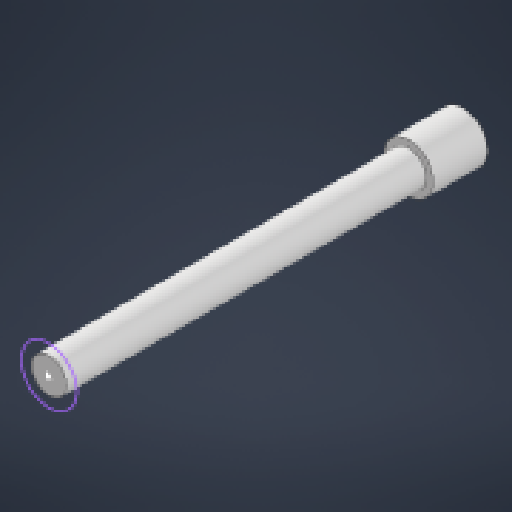
# Autodesk Inventor part: 丝杆
Saved by Autodesk Inventor 2025 (Build 290162000, 162)
## iProperties
Created: 2026-01-09
Part Number: 丝杆
Material: 常规
Document SubType Name: Modeling
Designer: XH
Density: 1 g/cm^3
Appearance: 默认
Author: XH
Autodesk Inventor part; units mm, degrees
ref_plane "YZ Plane" through (0, 0, 0) normal (1, 0, 0) x (0, 1, 0)
ref_plane "XZ Plane" through (0, 0, 0) normal (0, 1, 0) x (-1, 0, 0)
ref_plane "XY Plane" through (0, 0, 0) normal (0, 0, 1) x (1, 0, 0)
sketch "草图1" plane through (0, 0, 0) normal (0, 0, 1) x (1, 0, 0)
  circle A0 centre (0, 0) radius 1.5
  circle A1 centre (0, 0) radius 3.5
  dimension "d0" = 3
  dimension "d1" = 2
  constraints: 2 centre point, 2 coincident
  measures "d0" diameter of A0
  measures "d1" radial gap between concentric circles of A0 A1
extrude "拉伸1" add sketch "草图1" along normal blind 7.75
sketch "草图3" plane through (0, 0, 7.75) normal (0, 0, 1) x (1, 0, 0)
  circle A0 centre (0, 0) radius 3.5 projected
  circle A1 centre (0, 0) radius 1.5 projected
  circle A2 centre (0, 0) radius 2.5
  dimension "d4" = 1
  constraints: 1 centre point
  measures "d4" radial gap between concentric circles of A0 A2
extrude "拉伸2" add sketch "草图3" along normal blind 51.25 contours A1 | A2
sketch "草图5" plane through (0, 0, 0) normal (0, 1, 0) x (-1, 0, 0)
  line L0 (-3.3127, 60) -> (-1.5, 59)
  line L1 (2.5, 59) -> (-2.5, 59) projected
  line L2 (-1.5, 59) -> (-3.3127, 58)
  line L3 (-3.3127, 58) -> (-3.3127, 60)
  line L4 (-1.5, 59) -> (-3.3127, 59)
  point P0 (0, 0)
  dimension "d15" = 2
  dimension "d16" = 1
  constraints: 8 end point, 1 midpoint, 1 perpendicular, 1 point on line
  measures "d15" distance of L2.end L0.start
  measures "d16" distance of L1.end L0.end
coil "螺旋扫掠1" sketch "草图5" operation cut axis through (0, 0, -10) along (0, 0, -1) pitch 2.5 turns 20 hand right
